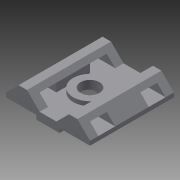
# Autodesk Inventor part: harness clip
Saved by Autodesk Inventor 2015 SP1 (Build 190203100, 203)
## iProperties
Created: 2015-02-19
Part Number: harness clip
Material: Generic
Document SubType Name: Modeling
Designer: Joseph
Density: 1 g/cm^3
Appearance: Default
Author: Joseph
Autodesk Inventor part; units mm, degrees
ref_plane "YZ Plane" through (0, 0, 0) normal (1, 0, 0) x (0, 1, 0)
ref_plane "XZ Plane" through (0, 0, 0) normal (0, 1, 0) x (-1, 0, 0)
ref_plane "XY Plane" through (0, 0, 0) normal (0, 0, 1) x (1, 0, 0)
sketch "Sketch1" plane through (0, 0, 0) normal (0, 0, 1) x (1, 0, 0)
  line L0 (10, 10) -> (-10, 10)
  line L1 (-10, 10) -> (-10, -10)
  line L2 (-10, -10) -> (10, -10)
  line L3 (10, -10) -> (10, 10)
  line L4 (10, 10) -> (-10, -10) construction
  line L5 (-10, 10) -> (10, -10) construction
  dimension "d0" = 20
  dimension "d1" = 20
  constraints: 12 end point, 2 parallel, 1 horizontal, 1 perpendicular
  measures "d0" distance of L2.end L1.end
  measures "d1" distance of L1.end L0.end
extrude "Extrusion1" add sketch "Sketch1" along normal blind 4
sketch "Sketch2" plane through (0, 0, 0) normal (0, 0, -1) x (-1, 0, 0)
  line L0 (2, 1.1547) -> (2, -1.1547) projected
  line L1 (2, -1.1547) -> (0, -2.3094) projected
  line L2 (0, -2.3094) -> (-2, -1.1547) projected
  line L3 (-2, -1.1547) -> (-2, 1.1547) projected
  line L4 (-2, 1.1547) -> (0, 2.3094) projected
  line L5 (0, 2.3094) -> (2, 1.1547) projected
  line L6 (10, -10) -> (-10, -10) projected
  line L7 (-2.75, 10) -> (2.75, 10)
  line L8 (2.75, 10) -> (2.75, -10)
  line L9 (2.75, -10) -> (-2.75, -10)
  line L10 (-2.75, -10) -> (-2.75, 10)
  line L11 (-2.75, 10) -> (2.75, -10) construction
  line L12 (2.75, 10) -> (-2.75, -10) construction
  point P0 (0, 0)
  dimension "d5" = 5.5
  constraints: 12 end point, 2 midpoint, 2 parallel, 1 horizontal, 1 perpendicular, 1 point on line
  measures "d5" distance of L8.end L9.end
extrude "Extrusion2" add sketch "Sketch2" along normal blind 1
sketch "Sketch3" plane through (0, 0, -1) normal (0, 0, -1) x (-1, 0, 0)
  line L0 (2, -1.1547) -> (0, -2.3094) projected
  line L1 (0, -2.3094) -> (-2, -1.1547) projected
  line L2 (-2, -1.1547) -> (-2, 1.1547) projected
  line L3 (-2, 1.1547) -> (0, 2.3094) projected
  line L4 (0, 2.3094) -> (2, 1.1547) projected
  line L5 (2, 1.1547) -> (2, -1.1547) projected
  line L6 (-2.75, 2.75) -> (2.75, 2.75)
  line L7 (2.75, 2.75) -> (2.75, -2.75)
  line L8 (2.75, -2.75) -> (-2.75, -2.75)
  line L9 (-2.75, -2.75) -> (-2.75, 2.75)
  line L10 (-2.75, 2.75) -> (2.75, -2.75) construction
  line L11 (2.75, 2.75) -> (-2.75, -2.75) construction
  point P0 (0, 0)
  dimension "d8" = 5.5
  dimension "d9" = 5.5
  constraints: 12 end point, 2 midpoint, 2 parallel, 1 horizontal, 1 perpendicular
  measures "d8" distance of L7.end L8.end
  measures "d9" distance of L6.end L7.end
extrude "Extrusion3" cut sketch "Sketch3" against normal up to surface (1 mm away) from surface at 0
sketch "Sketch4" plane through (10, -10, 0) normal (1, 0, 0) x (0, 0, -1)
  line L0 (-4, 0) -> (-4, 20) projected
  line L1 (0, 0) -> (-4, 0) projected
  line L2 (-3, 2) -> (-1, 2)
  line L3 (-1, 2) -> (-1, 6)
  line L4 (-1, 6) -> (-3, 6)
  line L5 (-3, 6) -> (-3, 2)
  line L6 (-3, 18) -> (-1, 18)
  line L7 (-1, 18) -> (-1, 14)
  line L8 (-1, 14) -> (-3, 14)
  line L9 (-3, 14) -> (-3, 18)
  circle A0 centre (-3, 0) radius 2 construction
  line L10 (0, 20) -> (-4, 20) projected
  line L11 (-3, 0) -> (-3, 20) construction
  circle A1 centre (-3, 20) radius 2 construction
  dimension "d35" = 4
  dimension "d31" = 2
  dimension "d32" = 4
  dimension "d33" = 2
  dimension "d34" = 4
  dimension "d36" = 1
  constraints: 18 end point, 4 parallel, 4 point on line, 3 perpendicular, 2 horizontal, 2 vertical alignment, 1 coincident, 4 other
  measures "d31" distance of L4.end L3.end
  measures "d32" distance of L3.end L2.end
  measures "d33" distance of L7.end L8.end
  measures "d34" distance of L6.end L7.end
  measures "d36" distance between parallel lines of L0 L5
extrude "Extrusion4" cut sketch "Sketch4" against normal up to surface (20 mm away) from surface at 0
sketch "Sketch6" plane through (0, 0, 4) normal (0, 0, 1) x (1, 0, 0)
  point P0 (0, 0)
  point P1 (0, 0)
  constraints: 1 coincident
hole "Hole1" at (0, 0, 4) direction (0, 0, -1) diameter 4.5 end through all counterbore diameter 8 counterbore depth 2
sketch "Sketch7" plane through (0, 0, 4) normal (0, 0, 1) x (1, 0, 0)
  circle A0 centre (0, 0) radius 4 projected
  line L0 (10, 10) -> (-10, 10) projected
  line L1 (-10, -10) -> (10, -10) projected
  line L2 (-4, 10) -> (4, 10)
  line L3 (4, 10) -> (4, -10)
  line L4 (4, -10) -> (-4, -10)
  line L5 (-4, -10) -> (-4, 10)
  line L6 (-4, 10) -> (4, -10) construction
  line L7 (4, 10) -> (-4, -10) construction
  line L8 (-10, -10) -> (-8, -10)
  line L9 (-8, -10) -> (-8, 10)
  line L10 (-8, 10) -> (-10, 10)
  line L11 (-10, 10) -> (-10, -10)
  line L12 (10, -10) -> (8, -10)
  line L13 (8, -10) -> (8, 10)
  line L14 (8, 10) -> (10, 10)
  line L15 (10, 10) -> (10, -10)
  dimension "d37" = 8
  dimension "d38" = 2
  dimension "d39" = 2
  constraints: 28 end point, 6 parallel, 3 horizontal, 3 perpendicular, 3 point on line, 2 midpoint
  measures "d37" distance between parallel lines of L3 L5
  measures "d38" distance of L10.end L9.end
  measures "d39" distance of L13.end L14.end
extrude "Extrusion6" cut sketch "Sketch7" against normal up to surface (3 mm away) from surface at 0 contours L3 L1 L5 A0 | A0 L5 L0 L3 | L0 L15 L1 L13 | L1 L11 L0 L9
chamfer "Chamfer1" distance 2 angle 45 3 edges at (-8, 0, 1) (-8, -9, 1) (-8, 9, 1)
chamfer "Chamfer2" distance 2 angle 45 3 edges at (8, 0, 1) (8, 9, 1) (8, -9, 1)
chamfer "Chamfer3" distance 1 angle 45 2 edges at (-8, 0, 4) (8, 0, 4)
chamfer "Chamfer4" distance 1 angle 45 4 edges at (4, -5, 4) (4, 5, 4) (-4, 5, 4) (-4, -5, 4)
chamfer "Chamfer5" distance 2 angle 45 2 edges at (4, 9, 1) (4, -9, 1)
chamfer "Chamfer6" distance 2 angle 45 2 edges at (-4, 9, 1) (-4, -9, 1)
body "Solid1"
